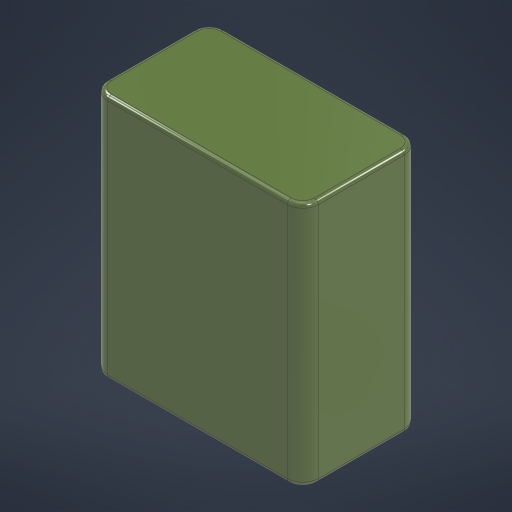
# Autodesk Inventor part: Battery Pack
Saved by Autodesk Inventor 2024 (Build 280153000, 153)
## iProperties
Created: 2025-11-11
Part Number: Battery Pack
Material: Generic
Document SubType Name: Modeling
Designer: Vincent Larson
Density: 1 g/cm^3
Appearance: Default
Author: Vincent Larson
Autodesk Inventor part; units mm, degrees
ref_plane "YZ Plane" through (0, 0, 0) normal (1, 0, 0) x (0, 1, 0)
ref_plane "XZ Plane" through (0, 0, 0) normal (0, 1, 0) x (-1, 0, 0)
ref_plane "XY Plane" through (0, 0, 0) normal (0, 0, 1) x (1, 0, 0)
sketch "Sketch1" plane through (0, 0, 0) normal (0, 1, 0) x (-1, 0, 0)
  line L0 (0, 0) -> (68.58, 0)
  line L1 (68.58, 0) -> (68.58, -38.1)
  line L2 (68.58, -38.1) -> (0, -38.1)
  line L3 (0, -38.1) -> (0, 0)
  dimension "d0" = 68.58
  dimension "d1" = 38.1
  constraints: 8 end point, 2 parallel, 1 horizontal, 1 perpendicular
  measures "d0" distance of L1.end L2.end
  measures "d1" distance of L0.end L1.end
extrude "Extrusion1" add sketch "Sketch1" along normal blind 79.756
fillet "Fillet1" radius 5.08 4 edges at (0, 39.878, 0) (0, 39.878, -38.1) (-68.58, 39.878, -38.1) (-68.58, 39.878, 0)
fillet "Fillet2" radius 1.27 16 edges at (-1.4879, 79.756, -1.4879) (0, 79.756, -19.05) (-1.4879, 79.756, -36.6121) (-34.29, 79.756, -38.1) (-67.0921, 79.756, -36.6121) (-68.58, 79.756, -19.05) (-67.0921, 79.756, -1.4879) (-34.29, 79.756, 0) (-1.4879, 0, -1.4879) (0, 0, -19.05) (-1.4879, 0, -36.6121) (-34.29, 0, -38.1) (-67.0921, 0, -36.6121) (-68.58, 0, -19.05) (-67.0921, 0, -1.4879) (-34.29, 0, 0)
body "Solid1"
